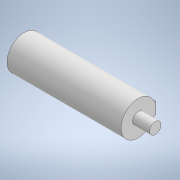
# Autodesk Inventor part: silnik_2
Saved by Autodesk Inventor 2022.3 (Build 263350000, 350)
## iProperties
Created: 2023-01-15
Part Number: silnik_2
Material: Generic
Document SubType Name: Modeling
Designer: komputer
Density: 1 g/cm^3
Appearance: Default
Author: komputer
Autodesk Inventor part; units mm, degrees
ref_plane "YZ Plane" through (0, 0, 0) normal (1, 0, 0) x (0, 1, 0)
ref_plane "XZ Plane" through (0, 0, 0) normal (0, 1, 0) x (-1, 0, 0)
ref_plane "XY Plane" through (0, 0, 0) normal (0, 0, 1) x (1, 0, 0)
sketch "Sketch1" plane through (0, 0, 0) normal (1, 0, 0) x (0, 1, 0)
  circle A0 centre (0, 0) radius 3
  dimension "d0" = 6
  constraints: 1 centre point, 1 coincident
  measures "d0" diameter of A0
extrude "Extrusion1" add sketch "Sketch1" along normal blind 20
sketch "Sketch2" plane through (20, 0, 0) normal (1, 0, 0) x (0, 0, -1)
  circle A0 centre (0, 0) radius 3 projected
  circle A1 centre (0, 0) radius 1
  dimension "d3" = 2
  constraints: 1 centre point, 1 coincident
  measures "d3" diameter of A1
extrude "Extrusion2" add sketch "Sketch2" along normal blind 3 contours A1
sketch "Sketch3" plane through (20, 0, 0) normal (1, 0, 0) x (0, 0, -1)
  circle A0 centre (0, 0) radius 1 projected
  circle A1 centre (0, 0) radius 3 projected
  line L0 (3, 0) -> (3.1, 0)
  line L1 (3.1, 0) -> (3.1, -1)
  line L2 (3.1, -1) -> (3.1, 1)
  line L3 (3.1, 1) -> (2.8284, 1)
  circle A2 centre (0, 0) radius 3 projected
  line L4 (3.1, -1) -> (2.8284, -1)
  dimension "d6" = 0.1
  dimension "d7" = 2
  constraints: 10 end point, 3 point on circle, 2 perpendicular, 1 horizontal, 1 parallel, 1 point on line
  measures "d6" distance of L0.start L0.end
  measures "d7" distance of L1.end L2.end
extrude "Extrusion3" add sketch "Sketch3" against normal up to surface (20 mm away) contours L0 L1 L4 A1 | A1 L3 L2 L0
body "Solid1"
